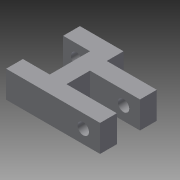
# Autodesk Inventor part: Pulley vice
Saved by Autodesk Inventor 2014 SP1 (Build 180222100, 222)
## iProperties
Created: 2014-07-08
Part Number: Pulley vice
Material: Generic
Document SubType Name: Modeling
Designer: Nick
Density: 1 g/cm^3
Appearance: Default
Author: Nick
Autodesk Inventor part; units mm, degrees
ref_plane "YZ Plane" through (0, 0, 0) normal (1, 0, 0) x (0, 1, 0)
ref_plane "XZ Plane" through (0, 0, 0) normal (0, 1, 0) x (-1, 0, 0)
ref_plane "XY Plane" through (0, 0, 0) normal (0, 0, 1) x (1, 0, 0)
sketch "Sketch1" plane through (0, 0, 0) normal (0, 0, 1) x (1, 0, 0)
  line L0 (0, 0) -> (15, 0)
  line L1 (15, 0) -> (15, -5)
  line L2 (15, -5) -> (-13, -5)
  line L3 (-13, -5) -> (-13, 0)
  line L4 (-13, 0) -> (-5, 0)
  line L5 (-5, 0) -> (-5, 12)
  line L6 (-5, 12) -> (-13, 12)
  line L7 (-13, 12) -> (-13, 17)
  line L8 (14.8978, 12) -> (14.8978, 7)
  line L9 (14.8978, 7) -> (0, 7)
  line L10 (0, 7) -> (0, 0)
  line L11 (-13, 17) -> (0, 17)
  line L12 (0, 17) -> (0, 12)
  line L13 (0, 12) -> (14.8978, 12)
  dimension "d0" = 15
  dimension "d1" = 5
  dimension "d2" = 28
  dimension "d3" = 5
  dimension "d4" = 8
  dimension "d5" = 12
  dimension "d6" = 8
  dimension "d7" = 5
  dimension "d9" = 5
  dimension "d19" = 5
  constraints: 28 end point, 9 parallel, 3 perpendicular, 1 collinear, 1 horizontal
  measures "d0" distance of L0.start L0.end
  measures "d1" distance of L0.end L1.end
  measures "d2" distance of L1.end L2.end
  measures "d3" distance of L2.end L3.end
  measures "d4" distance of L3.end L4.end
  measures "d5" distance of L4.end L5.end
  measures "d6" distance of L5.end L6.end
  measures "d7" distance of L6.end L7.end
  measures "d9" distance of L8.start L8.end
  measures "d19" distance of L11.end L12.end
extrude "Extrusion1" add sketch "Sketch1" along normal blind 8
sketch "Sketch3" plane through (-13, 17, 0) normal (0, 1, 0) x (1, 0, 0)
  line L0 (0, 0) -> (0, -8) projected
  line L1 (13, 0) -> (13, -8) projected
  circle A0 centre (23, -4) radius 1.7
  circle A1 centre (4, -4) radius 1.7
  point P0 (13, -4)
  point P1 (13, -4)
  dimension "d20" = 3.4
  dimension "d21" = 3.4
  dimension "d22" = 4
  dimension "d23" = 10
  constraints: 2 centre point, 2 horizontal alignment, 2 midpoint
  measures "d20" diameter of A0
  measures "d21" diameter of A1
  measures "d22" distance from line of L0 A1.centre
  measures "d23" distance from line of L1 A0.centre
extrude "Extrusion3" cut sketch "Sketch3" against normal blind 30
delete faces "Delete Face1" heal yes whole lump no faces at (-7.322, -3.3333, 4.2727)
body "Solid1"
